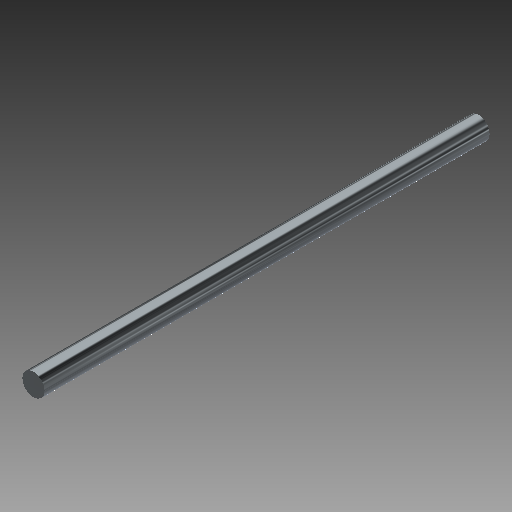
# Autodesk Inventor part: 275-1272
Saved by Autodesk Inventor 2018 (Build 220112000, 112)
## iProperties
Category: Structure
Company: Autodesk Inc.
Created: 2012-02-08
Part Number: 275-1272
Document SubType Name: Modeling
Designer: Autodesk Inc.
Density: 7.85 g/cm^3
Material: Steel
Catalog Web Link: http://www.vexrobotics.com/products/accessories/structure?ref=side
Vendor: VEX
Mass: 3.94658 g
Surface Area: 6.49219 cm^2
Volume: 0.502749 cm^3
Appearance: Zinc
Author: Autodesk Inc.
Autodesk Inventor part; units mm, degrees
ref_plane "YZ Plane" through (0, 0, 0) normal (1, 0, 0) x (0, 1, 0)
ref_plane "XZ Plane" through (0, 0, 0) normal (0, 1, 0) x (-1, 0, 0)
ref_plane "XY Plane" through (0, 0, 0) normal (0, 0, 1) x (1, 0, 0)
sketch "Sketch1" plane through (0, 0, 0) normal (0, 0, 1) x (1, 0, 0)
  circle A0 centre (0, 0) radius 1.5875
  dimension "d0" = 3.175
  constraints: 1 centre point, 1 coincident
  measures "d0" diameter of A0
extrude "Extrusion1" add sketch "Sketch1" against normal blind 63.5
body "Solid1"
